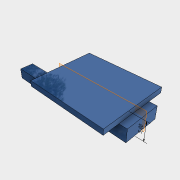
# Autodesk Inventor part: ЛЦМК0000002.00.00.00.00.03
Saved by Autodesk Inventor 2021.2 (Build 252289000, 289)
## iProperties
Created: 2025-10-23
Part Number: ЛЦМК0000002.00.00.00.00.03
Material: Типовые
Document SubType Name: Modeling
Designer: Захаров
Density: 1 g/cm^3
Appearance: С вкраплениями — сатинированная — синяя
Author: Захаров
Autodesk Inventor part; units mm, degrees
ref_plane "YZ Plane" through (0, 0, 0) normal (1, 0, 0) x (0, 1, 0)
ref_plane "XZ Plane" through (0, 0, 0) normal (0, 1, 0) x (-1, 0, 0)
ref_plane "РабПлоскость1" through (-8.75, -1.3, -1.3) normal (0, -1, 0) x (1, 0, 0)
sketch "Эскиз1" plane through (-8.75, -1.3, -1.3) normal (0, -1, 0) x (1, 0, 0)
  line L0 (21.5, -15.4) -> (0, -15.4)
  line L1 (0, -15.4) -> (0, 2.6)
  line L2 (0, 2.6) -> (21.5, 2.6)
  line L3 (21.5, 2.6) -> (21.5, -15.4)
  point P0 (8.75, 1.3)
  point P1 (0, 2.6)
  dimension "d0" = 21.5
  dimension "d1" = 18
  constraints: 8 end point, 2 parallel, 1 coincident, 1 horizontal, 1 perpendicular, 1 other
  measures "d0" distance of L1.end L2.end
  measures "d1" distance of L0.end L1.end
extrude "Выдавливание1" add sketch "Эскиз1" along normal blind 1.5
sketch "Эскиз2" plane through (-8.75, -2.8, -1.3) normal (0, -1, 0) x (1, 0, 0)
  line L0 (21.5, -15.4) -> (21.5, 2.6) projected
  line L1 (23.5, -1.65) -> (15, -1.65)
  line L2 (15, -1.65) -> (15, -11.15)
  line L3 (15, -11.15) -> (23.5, -11.15)
  line L4 (23.5, -11.15) -> (23.5, -1.65)
  point P0 (8.75, 1.3)
  point P1 (15, -6.4)
  point P2 (21.5, -6.4)
  dimension "d17" = 8.5
  dimension "d18" = 9.5
  dimension "d19" = 6.5
  constraints: 8 end point, 2 midpoint, 2 parallel, 1 horizontal, 1 horizontal alignment, 1 perpendicular
  measures "d17" distance of L3.end L2.end
  measures "d18" distance of L2.end L1.end
  measures "d19" distance between parallel lines of L2 L0
extrude "Выдавливание2" add sketch "Эскиз2" along normal blind 3.5
ref_plane "РабПлоскость2" through (-8.75, -1.3, -7.7) normal (0, 0, 1) x (1, 0, 0)
sketch "Эскиз4" plane through (-8.75, -2.8, -1.3) normal (0, -1, 0) x (1, 0, 0)
  line L0 (15, 0.35) -> (4, 0.35)
  line L1 (4, 0.35) -> (4, -13.15)
  line L2 (4, -13.15) -> (15, -13.15)
  line L3 (15, -13.15) -> (15, 0.35)
  line L4 (0, 2.6) -> (0, -15.4) projected
  point P0 (8.75, 1.3)
  point P1 (15, -6.4)
  point P2 (0, -6.4)
  dimension "d20" = 11
  dimension "d21" = 13.5
  dimension "d22" = 15
  constraints: 8 end point, 2 midpoint, 2 parallel, 1 horizontal, 1 horizontal alignment, 1 perpendicular
  measures "d20" distance of L2.end L1.end
  measures "d21" distance of L1.end L0.end
  measures "d22" distance between parallel lines of L4 L3
extrude "Выдавливание4" add sketch "Эскиз4" along normal blind 2.5
sketch "Эскиз5" plane through (-8.75, -2.8, -1.3) normal (0, -1, 0) x (1, 0, 0)
  line L0 (-1, -3.4) -> (4, -3.4)
  line L1 (4, -3.4) -> (4, 0.1)
  line L2 (4, 0.1) -> (-1, 0.1)
  line L3 (-1, 0.1) -> (-1, -3.4)
  line L4 (21.5, 2.6) -> (0, 2.6) projected
  line L5 (4, 0.35) -> (4, -13.15) projected
  point P0 (8.75, 1.3)
  point P1 (4, -1.65)
  point P2 (4, -6.4)
  dimension "d25" = 5
  dimension "d26" = 3.5
  dimension "d27" = 6
  constraints: 8 end point, 2 midpoint, 2 parallel, 1 horizontal, 1 perpendicular, 1 vertical alignment
  measures "d25" distance of L2.end L1.end
  measures "d26" distance of L1.end L0.end
  measures "d27" distance between parallel lines of L4 L0
extrude "Выдавливание5" add sketch "Эскиз5" along normal blind 2.6
sketch "Эскиз6" plane through (-9.75, -2.8, -4.7) normal (-1, 0, 0) x (0, 0, 1)
  circle A0 centre (1.75, -1.3) radius 1
  line L0 (3.5, -2.6) -> (0, -2.6) projected
  line L1 (3.5, 0) -> (3.5, -2.6) projected
  line L2 (3.5, 0) -> (0, 0) projected
  line L3 (0, 0) -> (0, -2.6) projected
  point P0 (4.7, 2.8)
  point P1 (1.75, -2.6)
  point P2 (3.5, -1.3)
  dimension "d30" = 2
  constraints: 2 midpoint, 1 centre point, 1 horizontal alignment, 1 vertical alignment
  measures "d30" diameter of A0
extrude "Выдавливание6" add sketch "Эскиз6" along normal blind 7 contours A0 | L0 L3 L2 L1
